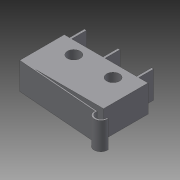
# Autodesk Inventor part: Micro Endstop Triggered
Saved by Autodesk Inventor 2015 SP1 (Build 190203100, 203)
## iProperties
Created: 2016-08-25
Part Number: Micro Endstop Triggered
Material: Generic
Document SubType Name: Modeling
Designer: Andrew
Density: 1 g/cm^3
Appearance: Default
Author: Andrew
Autodesk Inventor part; units mm, degrees
ref_plane "YZ Plane" through (0, 0, 0) normal (1, 0, 0) x (0, 1, 0)
ref_plane "XZ Plane" through (0, 0, 0) normal (0, 1, 0) x (-1, 0, 0)
ref_plane "XY Plane" through (0, 0, 0) normal (0, 0, 1) x (1, 0, 0)
sketch "Sketch1" plane through (0, 0, 0) normal (0, 0, 1) x (1, 0, 0)
  line L0 (0, 0) -> (19.75, 0)
  line L1 (19.75, 0) -> (19.75, 10.5)
  line L2 (0, 10.5) -> (0, 0)
  line L3 (1.2485, 10.5) -> (1.2485, 14)
  line L4 (1.2485, 14) -> (1.7485, 14)
  line L5 (1.7485, 14) -> (1.7485, 10.5)
  line L6 (9.135, 10.5) -> (9.135, 14)
  line L7 (9.135, 14) -> (9.635, 14)
  line L8 (9.635, 14) -> (9.635, 10.5)
  line L9 (17.5504, 10.5) -> (17.5504, 14)
  line L10 (17.5504, 14) -> (17.0504, 14)
  line L11 (17.0504, 14) -> (17.0504, 10.5)
  line L12 (19.75, 10.5) -> (17.5504, 10.5)
  line L13 (17.0504, 10.5) -> (9.635, 10.5)
  line L14 (9.135, 10.5) -> (1.7485, 10.5)
  line L15 (1.2485, 10.5) -> (0, 10.5)
  line L16 (5.25, 7.5) -> (14.5, 7.5) construction
  circle A0 centre (5.25, 7.5) radius 1.5
  circle A1 centre (14.5, 7.5) radius 1.5
  dimension "d0" = 19.75
  dimension "d1" = 10.5
  dimension "d2" = 14
  dimension "d3" = 0.5
  dimension "d6" = 3
  dimension "d7" = 3
  dimension "d8" = 5.25
  dimension "d9" = 5.25
  dimension "d17" = 9.25
  constraints: 34 end point, 23 perpendicular, 7 collinear, 5 parallel, 2 centre point, 2 coincident, 2 horizontal, 1 equal radius, 1 vertical
  measures "d0" distance of L0.start L0.end
  measures "d1" distance of L2.start L0.start
  measures "d2" distance between parallel lines of L0 L4
  measures "d3" distance of L3.end L4.end
  measures "d6" distance between parallel lines of L13 L16
  measures "d7" diameter of A0
  measures "d8" distance from line of L2 L16.start
  measures "d9" distance from line of L1 L16.end
  measures "d17" distance of L16.start L16.end
extrude "Extrusion1" add sketch "Sketch1" along normal blind 6.35
sketch "Sketch2" plane through (0, 0, 6.35) normal (0, 0, 1) x (1, 0, 0)
  line L0 (0, 0) -> (19.1921, -1.5105)
  line L1 (19.1921, -1.5105) -> (19.2157, -1.2105) construction
  line L2 (19.2157, -1.2105) -> (3.8355, 0)
  line L3 (0, 0) -> (19.75, 0) projected
  line L4 (0, 0) -> (3.8355, 0)
  arc A0 (19.1921, -1.5105) -> (22.3157, -1.4544) centre (20.7566, -1.6336) ccw
  line L5 (19.2157, -1.2105) -> (19.5157, -1.2341)
  line L6 (22.3157, -1.4544) -> (22.0157, -1.4308)
  arc A1 (19.5157, -1.2341) -> (22.0157, -1.4308) centre (20.75, -1.532) ccw
  line L7 (17.1531, -3.25) -> (26.6817, -3.25) construction
  line L8 (17.0504, 10.5) -> (9.635, 10.5) projected
  line L9 (19.75, 0) -> (19.75, 10.5) projected
  dimension "d10" = 0.3
  dimension "d11" = 13.75
  dimension "d12" = 4.5
  dimension "d13" = 2.5
  dimension "d14" = 1
  constraints: 14 end point, 4 point on circle, 3 collinear, 2 centre point, 2 equal length, 1 horizontal, 1 parallel, 1 perpendicular, 1 point on line, 1 tangent
  measures "d10" vertical distance of L0.end L1.end
  measures "d11" distance between parallel lines of L8 L7
  measures "d12" angle of L3 L2
  measures "d13" horizontal distance of L6.end L5.end
  measures "d14" distance from line of L9 A1.centre
extrude "Extrusion2" add sketch "Sketch2" against normal up to surface (6.35 mm away)
body "Solid1"
